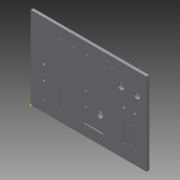
# Autodesk Inventor part: driver station 1.0
Saved by Autodesk Inventor 2015 (Build 190159000, 159)
## iProperties
Created: 2015-02-13
Part Number: driver station 1.0
Material: Generic
Document SubType Name: Modeling
Designer: szymsea16
Density: 1 g/cm^3
Appearance: Default
Author: szymsea16
Autodesk Inventor part; units mm, degrees
ref_plane "YZ Plane" through (0, 0, 0) normal (1, 0, 0) x (0, 1, 0)
ref_plane "XZ Plane" through (0, 0, 0) normal (0, 1, 0) x (-1, 0, 0)
ref_plane "XY Plane" through (0, 0, 0) normal (0, 0, 1) x (1, 0, 0)
sketch "Sketch1" plane through (0, 0, 0) normal (0, 0, 1) x (1, 0, 0)
  line L0 (0, 0) -> (419.1, 0)
  line L1 (419.1, 0) -> (419.1, 298.45)
  line L2 (419.1, 298.45) -> (0, 298.45)
  line L3 (0, 298.45) -> (0, 0)
  dimension "d0" = 419.1
  dimension "d1" = 298.45
  constraints: 8 end point, 2 parallel, 1 horizontal, 1 perpendicular
  measures "d0" distance of L2.end L1.end
  measures "d1" distance of L1.end L0.end
extrude "Extrusion1" add sketch "Sketch1" along normal blind 9.525
sketch "Sketch2" plane through (0, 0, 9.525) normal (0, 0, 1) x (1, 0, 0)
  line L0 (373.0625, 117.475) -> (376.2375, 117.475)
  line L1 (376.2375, 117.475) -> (376.2375, 47.625)
  line L2 (376.2375, 47.625) -> (373.0625, 47.625)
  line L3 (373.0625, 47.625) -> (373.0625, 117.475)
  line L4 (0, 0) -> (419.1, 0) projected
  line L5 (419.1, 0) -> (419.1, 298.45) projected
  circle A0 centre (374.65, 41.275) radius 1.5875
  circle A1 centre (374.65, 123.825) radius 1.5875
  circle A2 centre (374.65, 161.925) radius 5.08
  circle A3 centre (336.55, 41.275) radius 1.5875
  line L6 (338.1375, 47.625) -> (334.9625, 47.625)
  line L7 (334.9625, 47.625) -> (334.9625, 117.475)
  line L8 (334.9625, 117.475) -> (338.1375, 117.475)
  line L9 (338.1375, 117.475) -> (338.1375, 47.625)
  circle A4 centre (336.55, 123.825) radius 1.5875
  circle A5 centre (336.55, 161.925) radius 5.08
  circle A6 centre (383.8448, 222.25) radius 12.065
  circle A7 centre (325.4248, 222.25) radius 12.065
  line L10 (299.4225, 0) -> (299.4225, 298.45)
  dimension "d4" = 3.175
  dimension "d5" = 69.85
  dimension "d6" = 47.625
  dimension "d7" = 42.8625
  dimension "d8" = 3.175
  dimension "d9" = 6.35
  dimension "d10" = 3.175
  dimension "d11" = 6.35
  dimension "d12" = 10.16
  dimension "d13" = 38.1
  dimension "d16" = 3.175
  dimension "d17" = 38.1
  dimension "d18" = 69.85
  dimension "d19" = 3.175
  dimension "d20" = 10.16
  dimension "d23" = 24.13
  dimension "d24" = 35.2552
  dimension "d25" = 93.6752
  dimension "d26" = 58.42
  dimension "d27" = 60.325
  constraints: 18 end point, 8 centre point, 4 parallel, 2 horizontal, 2 perpendicular, 1 point on line, 1 vertical
  measures "d4" distance of L1.end L2.end
  measures "d5" distance of L0.end L1.end
  measures "d6" distance between parallel lines of L4 L2
  measures "d7" distance between parallel lines of L5 L1
  measures "d8" diameter of A0
  measures "d9" distance from line of A0.centre L2
  measures "d10" diameter of A1
  measures "d11" distance from line of L0 A1.centre
  measures "d12" diameter of A2
  measures "d13" distance of A1.centre A2.centre
  measures "d16" diameter of A3
  measures "d17" distance of A3.centre A0.centre
  measures "d18" distance of L6.end L7.end
  measures "d19" diameter of A4
  measures "d20" diameter of A5
  measures "d23" diameter of A6
  measures "d24" distance from line of L5 A6.centre
  measures "d25" distance from line of L5 A7.centre
  measures "d26" distance of A6.centre A7.centre
  measures "d27" vertical distance of A2.centre A6.centre
extrude "Extrusion2" cut sketch "Sketch2" against normal blind 9.525
sketch "Sketch3" plane through (0, 0, 9.525) normal (0, 0, 1) x (1, 0, 0)
  point P0 (0, 0)
sketch "Sketch4" plane through (0, 0, 9.525) normal (0, 0, 1) x (1, 0, 0)
  line L0 (419.1, 298.45) -> (0, 298.45) projected
  line L1 (287.3248, 298.45) -> (287.3248, 0)
  line L2 (0, 0) -> (419.1, 0) projected
  circle A0 centre (325.4248, 222.25) radius 12.065 projected
  line L3 (261.9248, 38.1) -> (192.0748, 38.1)
  line L4 (192.0748, 38.1) -> (192.0748, 41.275)
  line L5 (192.0748, 41.275) -> (261.9248, 41.275)
  line L6 (261.9248, 41.275) -> (261.9248, 38.1)
  circle A1 centre (185.7248, 39.6875) radius 1.5875
  circle A2 centre (268.2748, 39.6875) radius 1.5875
  circle A3 centre (249.2248, 95.25) radius 12.065
  circle A4 centre (198.4248, 95.25) radius 4.445
  circle A5 centre (198.4248, 146.05) radius 4.445
  dimension "d30" = 38.1
  dimension "d31" = 69.85
  dimension "d32" = 3.175
  dimension "d33" = 38.1
  dimension "d34" = 25.4
  dimension "d35" = 6.35
  dimension "d36" = 6.35
  dimension "d37" = 24.13
  dimension "d38" = 95.25
  dimension "d39" = 38.1
  dimension "d68" = 8.89
  dimension "d69" = 50.8
  dimension "d70" = 8.89
  dimension "d71" = 50.8
  constraints: 10 end point, 5 centre point, 2 parallel, 2 point on line, 1 horizontal, 1 perpendicular, 1 vertical
  measures "d30" distance from line of A0.centre L1
  measures "d31" distance of L4.end L5.end
  measures "d32" distance of L3.end L4.end
  measures "d33" distance between parallel lines of L2 L3
  measures "d34" distance between parallel lines of L1 L6
  measures "d35" distance from line of L4 A1.centre
  measures "d36" distance from line of A2.centre L6
  measures "d37" diameter of A3
  measures "d38" distance from line of L2 A3.centre
  measures "d39" distance from line of L1 A3.centre
  measures "d68" diameter of A4
  measures "d69" distance of A3.centre A4.centre
  measures "d70" diameter of A5
  measures "d71" distance of A4.centre A5.centre
extrude "Extrusion3" cut sketch "Sketch4" against normal blind 9.525 contours L3 L4 L5 L6 | A1 | A2 | A3 | A4 | A5
sketch "Sketch5" plane through (0, 0, 9.525) normal (0, 0, 1) x (1, 0, 0)
  line L0 (0, 0) -> (419.1, 0) projected
  line L1 (147.6248, 0) -> (147.6248, 296.9243)
  line L2 (261.9248, 41.275) -> (261.9248, 38.1) projected
  line L3 (104.1241, 107.95) -> (107.2991, 107.95)
  line L4 (107.2991, 107.95) -> (107.2991, 38.1)
  line L5 (107.2991, 38.1) -> (104.1241, 38.1)
  line L6 (104.1241, 38.1) -> (104.1241, 107.95)
  circle A0 centre (105.7116, 31.75) radius 1.5875
  circle A1 centre (105.7116, 114.3) radius 1.5875
  circle A2 centre (46.0248, 101.6) radius 5.08
  circle A3 centre (46.0248, 38.1) radius 3.048
  line L7 (419.1, 298.45) -> (0, 298.45) projected
  line L8 (292.8764, 298.45) -> (292.8764, 0)
  circle A4 centre (46.0248, 152.4) radius 4.7625
  dimension "d42" = 114.3
  dimension "d43" = 3.175
  dimension "d44" = 69.85
  dimension "d45" = 38.1
  dimension "d46" = 3.175
  dimension "d47" = 6.35
  dimension "d48" = 3.175
  dimension "d49" = 6.35
  dimension "d50" = 10.16
  dimension "d51" = 101.6
  dimension "d52" = 101.6
  dimension "d53" = 6.096
  dimension "d72" = 9.525
  dimension "d73" = 50.8
  constraints: 12 end point, 5 centre point, 3 point on line, 2 parallel, 2 perpendicular, 1 horizontal, 1 vertical
  measures "d42" distance between parallel lines of L2 L1
  measures "d43" distance of L4.end L5.end
  measures "d44" distance of L3.end L4.end
  measures "d45" distance between parallel lines of L0 L5
  measures "d46" diameter of A0
  measures "d47" vertical distance of L4.end A0.centre
  measures "d48" diameter of A1
  measures "d49" distance from line of L3 A1.centre
  measures "d50" diameter of A2
  measures "d51" distance from line of L1 A2.centre
  measures "d52" distance from line of L0 A2.centre
  measures "d53" diameter of A3
  measures "d72" diameter of A4
  measures "d73" distance of A2.centre A4.centre
sketch "Sketch6" plane through (0, 0, 9.525) normal (0, 0, 1) x (1, 0, 0)
  line L0 (0, 222.25) -> (296.6633, 222.25)
  line L1 (419.1, 298.45) -> (0, 298.45) projected
  circle A0 centre (101.6, 260.35) radius 3.048
  line L2 (0, 298.45) -> (0, 0) projected
  circle A1 centre (152.4, 260.35) radius 3.048
  circle A2 centre (203.2, 260.35) radius 3.048
  circle A3 centre (292.1, 260.35) radius 3.048
  dimension "d54" = 76.2
  dimension "d55" = 6.096
  dimension "d56" = 101.6
  dimension "d57" = 38.1
  dimension "d58" = 6.096
  dimension "d59" = 50.8
  dimension "d60" = 6.096
  dimension "d61" = 50.8
  dimension "d62" = 6.096
  dimension "d63" = 88.9
  constraints: 4 centre point, 2 end point, 1 horizontal
  measures "d54" distance between parallel lines of L0 L1
  measures "d55" diameter of A0
  measures "d56" distance from line of L2 A0.centre
  measures "d57" distance from line of L0 A0.centre
  measures "d58" diameter of A1
  measures "d59" distance of A1.centre A0.centre
  measures "d60" diameter of A2
  measures "d61" distance of A2.centre A1.centre
  measures "d62" diameter of A3
  measures "d63" distance of A3.centre A2.centre
extrude "Extrusion4" cut sketch "Sketch5" against normal blind 9.525
extrude "Extrusion5" cut sketch "Sketch6" against normal blind 9.525
body "Solid1"
